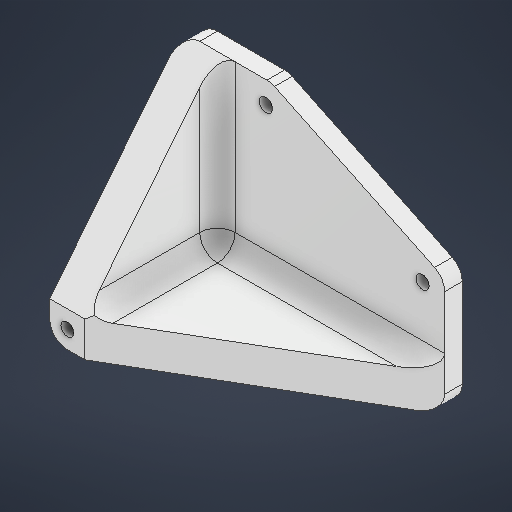
# Autodesk Inventor part: FrontLevelBlock
Saved by Autodesk Inventor 2026.2 (Build 302298000, 298)
## iProperties
Created: 2026-06-02
Part Number: FrontLevelBlock
Material: ABS Plastic
Document SubType Name: Modeling
Designer: gaoet
Density: 1.06 g/cm^3
Appearance: Smooth - White
Author: gaoet
Autodesk Inventor part; units mm, degrees
ref_plane "YZ Plane" through (0, 0, 0) normal (1, 0, 0) x (0, 1, 0)
ref_plane "XZ Plane" through (0, 0, 0) normal (0, 1, 0) x (-1, 0, 0)
ref_plane "XY Plane" through (0, 0, 0) normal (0, 0, 1) x (1, 0, 0)
sketch "Sketch1" plane through (0, 0, 0) normal (0, 0, 1) x (1, 0, 0)
  line L0 (-19, 5) -> (40.5, 5)
  line L1 (40.5, 5) -> (40.5, -40.5)
  line L2 (40.5, -40.5) -> (-19, -40.5)
  line L3 (-19, -40.5) -> (-19, 5)
  line L4 (1.1354, 5) -> (40.5, -13.8506)
  line L5 (35.5, -17) -> (0, 0) construction
  point P0 (-15, -36.5)
  dimension "d0" = 35.5
  dimension "d1" = 17
  dimension "d2" = 50.5
  dimension "d3" = 19.5
  dimension "d4" = 5
  dimension "d5" = 5
  dimension "d6" = 4
  dimension "d7" = 4
  dimension "d31" = 5
  constraints: 12 end point, 3 parallel, 2 point on line, 1 coincident, 1 horizontal, 1 perpendicular
  measures "d0" horizontal distance of L5.start point (0, 0)
  measures "d1" vertical distance of point (0, 0) L5.start
  measures "d2" horizontal distance of L5.start point (-15, -36.5)
  measures "d3" vertical distance of L5.start point (-15, -36.5)
  measures "d4" distance from line of L0 point (0, 0)
  measures "d5" distance from line of L1 L5.start
  measures "d6" distance from line of L3 point (-15, -36.5)
  measures "d7" distance from line of L2 point (-15, -36.5)
  measures "d31" distance between parallel lines of L5 L4
extrude "Extrusion1" add sketch "Sketch1" along normal blind 4 contours L0 L4 L1 L2 L3
hole "Hole1" at (35.5, -17, 0) at (0, 0, 0) direction (0, 0, 1) diameter 3 depth 20
sketch "Sketch2" plane through (-19, -40.5, 0) normal (0, -1, 0) x (1, 0, 0)
  line L0 (0, 0) -> (59.5, 0) projected
  line L1 (59.5, 0) -> (59.5, 4) projected
  line L2 (0, 4) -> (59.5, 4) projected
  line L3 (0, 0) -> (0, 4) projected
  line L4 (0, 4) -> (0, 34)
  line L5 (0, 34) -> (8, 34)
  line L6 (8, 34) -> (59.5, 4)
  point P0 (19, 0)
  dimension "d17" = 34
  dimension "d18" = 8
  constraints: 6 end point, 1 horizontal, 1 vertical
  measures "d17" distance between parallel lines of L0 L5
  measures "d18" distance of L4.end L5.end
extrude "Extrusion2" add sketch "Sketch2" against normal blind 8 contours L4 L5 L6 L2
sketch "Sketch3" plane through (-19, -40.5, 0) normal (-1, 0, 0) x (0, 0, 1)
  line L0 (0, 45.5) -> (0, 0) projected
  line L1 (0, 0) -> (34, 0) projected
  line L2 (34, 0) -> (34, 8) projected
  line L3 (4, 8) -> (34, 8) projected
  line L4 (4, 45.5) -> (4, 8) projected
  line L5 (0, 45.5) -> (4, 45.5) projected
  line L6 (34, 8) -> (4, 45.5)
  point P0 (0, 40.5)
  constraints: 2 end point
extrude "Extrusion3" add sketch "Sketch3" against normal blind 8 contours L6 L3 L4
fillet "Fillet1" radius 4 8 edges at (-11, -13.75, 4) (14.75, -32.5, 4) (-11, -32.5, 19) (40.5, -40.5, 2) (-19, 5, 2) (1.1354, 5, 2) (40.5, -13.8506, 2) (-19, -40.5, 17)
sketch "Sketch4" plane through (-19, -40.5, 34) normal (0, 0, 1) x (1, 0, 0)
  line L0 (8, 0) -> (4, 0) projected
  line L1 (8, 0) -> (8, 8) projected
  line L2 (0, 8) -> (8, 8) projected
  line L3 (0, 4) -> (0, 8) projected
  arc A0 (0, 4) -> (4, 0) centre (4, 4) ccw projected
  point P0 (19, 40.5)
  point P1 (4, 4)
hole "Hole2" at (-15, -36.5, 34) direction (0, 0, -1) diameter 2.9 depth 20
equation "\"d5\" = d4"
equation "\"d6\" = d7"
equation "\"d23\" = d7"
body "Solid1"
